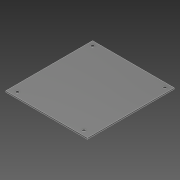
# Autodesk Inventor part: pc104standard
Saved by Autodesk Inventor 2020 (Build 240168000, 168)
## iProperties
Created: 2021-04-30
Part Number: pc104standard
Material: Generic
Document SubType Name: Modeling
Designer: Bowen O'Steen
Density: 1 g/cm^3
Appearance: Smooth - Black
Author: Bowen O'Steen
Autodesk Inventor part; units mm, degrees
ref_plane "YZ Plane" through (0, 0, 0) normal (1, 0, 0) x (0, 1, 0)
ref_plane "XZ Plane" through (0, 0, 0) normal (0, 1, 0) x (-1, 0, 0)
ref_plane "XY Plane" through (0, 0, 0) normal (0, 0, 1) x (1, 0, 0)
sketch "Sketch1" plane through (0, 0, 0) normal (0, 1, 0) x (-1, 0, 0)
  line L0 (45.085, 47.945) -> (-45.085, 47.945)
  line L1 (-45.085, 47.945) -> (-45.085, -47.945)
  line L2 (-45.085, -47.945) -> (45.085, -47.945)
  line L3 (45.085, -47.945) -> (45.085, 47.945)
  point P0 (0, 0)
  point P1 (0, -47.945)
  point P2 (45.085, 0)
  dimension "d0" = 95.89
  dimension "d1" = 90.17
  constraints: 8 end point, 2 midpoint, 2 parallel, 1 horizontal, 1 horizontal alignment, 1 perpendicular, 1 vertical alignment
  measures "d0" distance of L2.end L0.start
  measures "d1" distance of L1.end L2.end
extrude "Extrusion1" add sketch "Sketch1" along normal blind 1.57
sketch "Sketch2" plane through (0, 1.57, 0) normal (0, 1, 0) x (1, 0, 0)
  line L0 (0, 0) -> (0, 7.4645) construction
  line L1 (45.085, 47.945) -> (-45.085, 47.945) projected
  line L2 (45.085, -47.945) -> (45.085, 47.945) projected
  point P0 (-40.005, 42.865)
  point P1 (-37.465, -42.865)
  point P2 (40.005, 42.865)
  point P3 (36.195, -42.865)
  dimension "d5" = 85.09
  dimension "d6" = 5.08
  dimension "d7" = 82.55
  dimension "d8" = 90.81
  dimension "d16" = 8.89
  dimension "d17" = 90.81
  dimension "d18" = 5.08
  dimension "d19" = 5.08
  constraints: 2 end point, 1 vertical
  measures "d5" distance from line of L2 point (-40.005, 42.865)
  measures "d6" distance from line of L1 point (-40.005, 42.865)
  measures "d7" distance from line of L2 point (-37.465, -42.865)
  measures "d8" distance from line of L1 point (-37.465, -42.865)
  measures "d16" distance from line of L2 point (36.195, -42.865)
  measures "d17" distance from line of L1 point (36.195, -42.865)
  measures "d18" distance from line of L2 point (40.005, 42.865)
  measures "d19" distance from line of L1 point (40.005, 42.865)
hole "Hole1" at (-40.005, 1.57, -42.865) at (-37.465, 1.57, 42.865) at (36.195, 1.57, 42.865) at (40.005, 1.57, -42.865) direction (0, -1, 0) diameter 3.18 end through all
body "Solid1"
